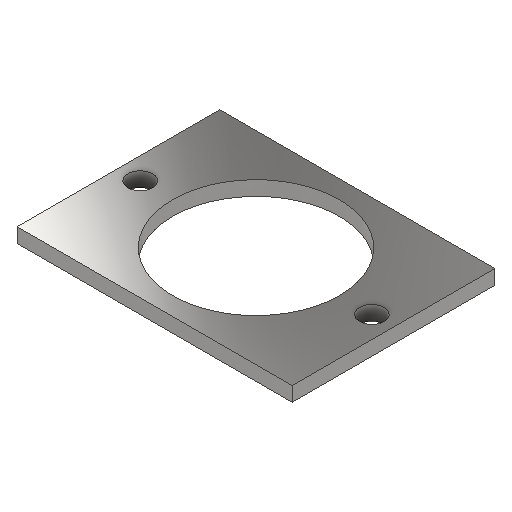
# Autodesk Inventor part: HayashiProbeHead_up
Saved by Autodesk Inventor 2026.2 (Build 302298000, 298)
## iProperties
Created: 2026-08-31
Part Number: HayashiProbeHead_up
Material: ステンレス鋼 440C
Document SubType Name: Modeling
Designer: zetsu
Density: 7.75 g/cm^3
Appearance: 半つや出し
Author: zetsu
Autodesk Inventor part; units mm, degrees
ref_plane "YZ Plane" through (0, 0, 0) normal (1, 0, 0) x (0, 1, 0)
ref_plane "XZ Plane" through (0, 0, 0) normal (0, 1, 0) x (-1, 0, 0)
ref_plane "XY Plane" through (0, 0, 0) normal (0, 0, 1) x (1, 0, 0)
sketch "スケッチ1" plane through (0, 0, 0) normal (0, 1, 0) x (-1, 0, 0)
  line L0 (19, -14) -> (-19, -14)
  line L1 (-19, -14) -> (-19, 14)
  line L2 (-19, 14) -> (19, 14)
  line L3 (19, 14) -> (19, -14)
  line L4 (0, -27.2114) -> (0, 0) construction
  line L5 (0, 0) -> (-35.5982, 0) construction
  dimension "d0" = 28
  dimension "d1" = 38
  constraints: 12 end point, 2 parallel, 2 perpendicular, 1 horizontal, 1 vertical, 2 other
  measures "d0" distance of L2.end L0.start
  measures "d1" distance of L1.end L2.end
extrude "押し出し1" add sketch "スケッチ1" along normal blind 2
sketch "スケッチ2" plane through (0, 2, 0) normal (0, 1, 0) x (1, 0, 0)
  circle A0 centre (0, 0) radius 11.5
  circle A1 centre (-16, 0) radius 1.7
  circle A2 centre (16, 0) radius 1.7
  line L0 (-19, 14) -> (-19, -14) projected
  line L1 (19, -14) -> (19, 14) projected
  dimension "d4" = 23
  dimension "d5" = 3.4
  dimension "d6" = 3.4
  dimension "d7" = 3
  dimension "d8" = 3
  constraints: 3 centre point, 1 coincident
  measures "d4" diameter of A0
  measures "d5" diameter of A1
  measures "d6" diameter of A2
  measures "d7" distance from line of A1.centre L0
  measures "d8" distance from line of L1 A2.centre
extrude "押し出し2" cut sketch "スケッチ2" against normal through all
